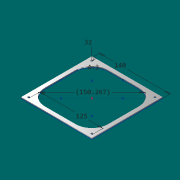
# Autodesk Inventor part: mesh_140
Saved by Autodesk Inventor 2022 (Build 260153000, 153)
## iProperties
Created: 2022-10-02
Part Number: mesh_140
Material: アルミニウム 6061
Document SubType Name: Modeling
Designer: gisen
Density: 2.7 g/cm^3
Appearance: アルミニウム - フラット
Author: gisen
Autodesk Inventor part; units mm, degrees
ref_plane "YZ Plane" through (0, 0, 0) normal (1, 0, 0) x (0, 1, 0)
ref_plane "XZ Plane" through (0, 0, 0) normal (0, 1, 0) x (-1, 0, 0)
ref_plane "XY Plane" through (0, 0, 0) normal (0, 0, 1) x (1, 0, 0)
sketch "スケッチ1" plane through (0, 0, 0) normal (0, 0, 1) x (1, 0, 0)
  line L0 (-70, 70) -> (70, 70)
  line L1 (70, 70) -> (70, -70)
  line L2 (70, -70) -> (-70, -70)
  line L3 (-70, -70) -> (-70, 70)
  line L4 (-62.5, 62.5) -> (62.5, 62.5) construction
  line L5 (62.5, 62.5) -> (62.5, -62.5) construction
  line L6 (62.5, -62.5) -> (-62.5, -62.5) construction
  line L7 (-62.5, -62.5) -> (-62.5, 62.5) construction
  circle A0 centre (-62.5, 62.5) radius 2.15
  line L8 (-30.5, 62.5) -> (30.5, 62.5)
  line L9 (62.5, 30.5) -> (62.5, -30.5)
  line L10 (30.5, -62.5) -> (-30.5, -62.5)
  line L11 (-62.5, -30.5) -> (-62.5, 30.5)
  arc A1 (-30.5, 62.5) -> (-62.5, 30.5) centre (-30.5, 30.5) ccw
  arc A2 (-62.5, -30.5) -> (-30.5, -62.5) centre (-30.5, -30.5) ccw
  arc A3 (30.5, -62.5) -> (62.5, -30.5) centre (30.5, -30.5) ccw
  arc A4 (62.5, 30.5) -> (30.5, 62.5) centre (30.5, 30.5) ccw
  line L12 (53.1274, 53.1274) -> (-53.1274, -53.1274) construction
  circle A5 centre (-62.5, -62.5) radius 2.15
  circle A6 centre (62.5, -62.5) radius 2.15
  circle A7 centre (62.5, 62.5) radius 2.15
  point P0 (0, 0)
  point P1 (-70, 0)
  point P2 (0, 70)
  point P3 (-62.5, 0)
  point P4 (0, 62.5)
  dimension "d0" = 140
  dimension "d1" = 125
  dimension "d3" = 4.3
  dimension "d4" = 32
  dimension "d5" = 150.267
  constraints: 26 end point, 10 point on circle, 8 centre point, 8 tangent, 6 equal radius, 6 midpoint, 6 parallel, 5 perpendicular, 4 coincident, 3 horizontal, 2 horizontal alignment, 2 point on line, 2 vertical alignment
  measures "d0" distance of L0.start L0.end
  measures "d1" distance of L5.end L6.end
  measures "d3" diameter of A0
  measures "d4" radius of A1
  measures "d5" distance of L12.start L12.end
extrude "押し出し1" add sketch "スケッチ1" along normal blind 2.2
